Autodesk Inventor part; units mm, degrees
(part 2 of 3)
  spline S109 degree 2 poles (-64.4838, -130.0747) (-64.4838, -130.0909) (-64.4903, -130.1136) knots 0 0 0 1 1 1
  line L121 (-64.4903, -130.1136) -> (-65.1883, -133.2532)
  spline S110 degree 2 poles (-65.1883, -133.2532) (-65.2175, -133.3994) (-65.3604, -133.3994) knots 0 0 0 1 1 1
  spline S111 degree 2 poles (-65.3604, -133.3994) (-65.4838, -133.3994) (-65.5357, -133.2468) knots 0 0 0 1 1 1
  line L122 (-65.5357, -133.2468) -> (-66.0584, -131.6753)
  line L123 (-66.0584, -131.6753) -> (-66.5812, -133.2468)
  spline S112 degree 2 poles (-66.5812, -133.2468) (-66.6331, -133.3994) (-66.7597, -133.3994) knots 0 0 0 1 1 1
  spline S113 degree 2 poles (-66.7597, -133.3994) (-66.8961, -133.3994) (-66.9318, -133.2468) knots 0 0 0 1 1 1
  line L124 (-66.9318, -133.2468) -> (-67.6299, -130.1136)
  spline S114 degree 2 poles (-67.6299, -130.1136) (-67.6331, -130.0909) (-67.6331, -130.0747) knots 0 0 0 1 1 1
  spline S115 degree 2 poles (-67.6331, -130.0747) (-67.6331, -129.8994) (-67.4578, -129.8994) knots 0 0 0 1 1 1
  spline S116 degree 2 poles (-67.4578, -129.8994) (-67.3182, -129.8994) (-67.2857, -130.0357) knots 0 0 0 1 1 1
  line L125 (-67.2857, -130.0357) -> (-66.724, -132.5714)
  line L126 (-66.724, -132.5714) -> (-66.2305, -131.0942)
  spline S117 degree 2 poles (-66.2305, -131.0942) (-66.1851, -130.9513) (-66.0584, -130.9513) knots 0 0 0 1 1 1
  spline S118 degree 2 poles (-66.0584, -130.9513) (-65.9318, -130.9513) (-65.8831, -131.0942) knots 0 0 0 1 1 1
  line L127 (-65.8831, -131.0942) -> (-65.3929, -132.5682)
  spline S119 degree 2 poles (-62.9123, -133.3994) (-63.276, -133.3994) (-63.7857, -132.8864) (-63.7857, -132.5227) knots 0 0 0 1 2 2 2
  line L128 (-63.7857, -132.5227) -> (-63.7857, -132.1753)
  spline S120 degree 2 poles (-63.7857, -132.1753) (-63.7857, -131.7403) (-63.4351, -131.474) knots 0 0 0 1 1 1
  spline S121 degree 2 poles (-63.4351, -131.474) (-63.7857, -131.2078) (-63.7857, -130.7727) knots 0 0 0 1 1 1
  spline S122 degree 2 poles (-63.7857, -130.7727) (-63.7857, -130.4123) (-63.276, -129.8994) (-62.9123, -129.8994) knots 0 0 0 1 2 2 2
  spline S123 degree 2 poles (-62.9123, -129.8994) (-62.5487, -129.8994) (-62.039, -130.4123) (-62.039, -130.7727) knots 0 0 0 1 2 2 2
  spline S124 degree 2 poles (-62.039, -130.7727) (-62.039, -131.2078) (-62.3896, -131.474) knots 0 0 0 1 1 1
  spline S125 degree 2 poles (-62.3896, -131.474) (-62.1364, -131.6656) (-62.0714, -131.9448) knots 0 0 0 1 1 1
  spline S126 degree 2 poles (-62.0714, -131.9448) (-62.039, -132.0844) (-62.039, -132.5227) knots 0 0 0 1 1 1
  spline S127 degree 2 poles (-62.039, -132.5227) (-62.039, -132.8864) (-62.5487, -133.3994) (-62.9123, -133.3994) knots 0 0 0 1 2 2 2
  spline S128 degree 2 poles (-62.9123, -133.0487) (-62.6948, -133.0487) (-62.3896, -132.7435) (-62.3896, -132.5227) knots 0 0 0 1 2 2 2
  line L129 (-62.3896, -132.5227) -> (-62.3896, -132.1753)
  spline S129 degree 2 poles (-62.3896, -132.1753) (-62.3896, -131.9578) (-62.6948, -131.6494) (-62.9123, -131.6494) knots 0 0 0 1 2 2 2
  spline S130 degree 2 poles (-62.9123, -131.6494) (-63.1299, -131.6494) (-63.4351, -131.9545) (-63.4351, -132.1753) knots 0 0 0 1 2 2 2
  line L130 (-63.4351, -132.1753) -> (-63.4351, -132.5227)
  spline S131 degree 2 poles (-63.4351, -132.5227) (-63.4351, -132.7435) (-63.1299, -133.0487) (-62.9123, -133.0487) knots 0 0 0 1 2 2 2
  spline S132 degree 2 poles (-62.9123, -131.2987) (-62.6948, -131.2987) (-62.3896, -130.9968) (-62.3896, -130.776) knots 0 0 0 1 2 2 2
  spline S133 degree 2 poles (-62.3896, -130.776) (-62.3896, -130.5584) (-62.6948, -130.25) (-62.9123, -130.25) knots 0 0 0 1 2 2 2
  spline S134 degree 2 poles (-62.9123, -130.25) (-63.1299, -130.25) (-63.4351, -130.5552) (-63.4351, -130.776) knots 0 0 0 1 2 2 2
  spline S135 degree 2 poles (-63.4351, -130.776) (-63.4351, -130.9968) (-63.1299, -131.2987) (-62.9123, -131.2987) knots 0 0 0 1 2 2 2
  spline S136 degree 2 poles (-60.8117, -133.3994) (-60.8799, -133.3994) (-60.987, -133.2922) (-60.987, -133.224) knots 0 0 0 1 2 2 2
  spline S137 degree 2 poles (-60.987, -133.224) (-60.987, -133.1039) (-60.8994, -133.0747) knots 0 0 0 1 1 1
  spline S138 degree 2 poles (-60.8994, -133.0747) (-60.711, -133.0097) (-60.5844, -132.9286) knots 0 0 0 1 1 1
  spline S139 degree 2 poles (-60.5844, -132.9286) (-60.0195, -132.5617) (-59.9545, -132) knots 0 0 0 1 1 1
  line L131 (-59.9545, -132) -> (-60.4643, -132)
  spline S140 degree 2 poles (-60.4643, -132) (-60.8279, -132) (-61.3377, -131.487) (-61.3377, -131.1234) knots 0 0 0 1 2 2 2
  line L132 (-61.3377, -131.1234) -> (-61.3377, -130.776)
  spline S141 degree 2 poles (-61.3377, -130.776) (-61.3377, -130.4123) (-60.8279, -129.8994) (-60.4643, -129.8994) knots 0 0 0 1 2 2 2
  spline S142 degree 2 poles (-60.4643, -129.8994) (-60.1006, -129.8994) (-59.5909, -130.4058) (-59.5909, -130.7695) knots 0 0 0 1 2 2 2
  line L133 (-59.5909, -130.7695) -> (-59.5909, -131.8247)
  spline S143 degree 2 poles (-59.5909, -131.8247) (-59.5909, -132.7143) (-60.4188, -133.2338) knots 0 0 0 1 1 1
  spline S144 degree 2 poles (-60.4188, -133.2338) (-60.6851, -133.3994) (-60.8117, -133.3994) knots 0 0 0 1 1 1
  line L134 (-59.9416, -131.6494) -> (-59.9416, -130.776)
  spline S145 degree 2 poles (-59.9416, -130.776) (-59.9416, -130.5584) (-60.2468, -130.25) (-60.4643, -130.25) knots 0 0 0 1 2 2 2
  spline S146 degree 2 poles (-60.4643, -130.25) (-60.6818, -130.25) (-60.987, -130.5584) (-60.987, -130.776) knots 0 0 0 1 2 2 2
  line L135 (-60.987, -130.776) -> (-60.987, -131.1234)
  spline S147 degree 2 poles (-60.987, -131.1234) (-60.987, -131.3442) (-60.6818, -131.6494) (-60.4643, -131.6494) knots 0 0 0 1 2 2 2
  line L136 (-60.4643, -131.6494) -> (-59.9416, -131.6494)
  spline S148 degree 2 poles (-57.1429, -131.6494) (-57.1429, -132.276) (-57.2955, -132.7305) knots 0 0 0 1 1 1
  spline S149 degree 2 poles (-57.2955, -132.7305) (-57.5227, -133.3994) (-58.0162, -133.3994) knots 0 0 0 1 1 1
  spline S150 degree 2 poles (-58.0162, -133.3994) (-58.5097, -133.3994) (-58.737, -132.7338) knots 0 0 0 1 1 1
  spline S151 degree 2 poles (-58.737, -132.7338) (-58.8896, -132.2792) (-58.8896, -131.6494) knots 0 0 0 1 1 1
  spline S152 degree 2 poles (-58.8896, -131.6494) (-58.8896, -131.0195) (-58.737, -130.5649) knots 0 0 0 1 1 1
  spline S153 degree 2 poles (-58.737, -130.5649) (-58.5097, -129.8994) (-58.0162, -129.8994) knots 0 0 0 1 1 1
  spline S154 degree 2 poles (-58.0162, -129.8994) (-57.5227, -129.8994) (-57.2955, -130.5682) knots 0 0 0 1 1 1
  spline S155 degree 2 poles (-57.2955, -130.5682) (-57.1429, -131.0227) (-57.1429, -131.6494) knots 0 0 0 1 1 1
  spline S156 degree 2 poles (-57.4935, -131.6494) (-57.4935, -131.2143) (-57.5844, -130.8312) knots 0 0 0 1 1 1
  spline S157 degree 2 poles (-57.5844, -130.8312) (-57.7273, -130.25) (-58.0162, -130.25) knots 0 0 0 1 1 1
  spline S158 degree 2 poles (-58.0162, -130.25) (-58.3052, -130.25) (-58.4448, -130.8344) knots 0 0 0 1 1 1
  spline S159 degree 2 poles (-58.4448, -130.8344) (-58.539, -131.224) (-58.539, -131.6494) knots 0 0 0 1 1 1
  spline S160 degree 2 poles (-58.539, -131.6494) (-58.539, -132.0812) (-58.4481, -132.4675) knots 0 0 0 1 1 1
  spline S161 degree 2 poles (-58.4481, -132.4675) (-58.3052, -133.0487) (-58.0162, -133.0487) knots 0 0 0 1 1 1
  spline S162 degree 2 poles (-58.0162, -133.0487) (-57.7273, -133.0487) (-57.5844, -132.4675) knots 0 0 0 1 1 1
  spline S163 degree 2 poles (-57.5844, -132.4675) (-57.4935, -132.0812) (-57.4935, -131.6494) knots 0 0 0 1 1 1
  line L137 (-54.8669, -132.526) -> (-56.2662, -132.526)
  spline S164 degree 2 poles (-56.2662, -132.526) (-56.4416, -132.526) (-56.4416, -132.3506) knots 0 0 0 1 1 1
  spline S165 degree 2 poles (-56.4416, -132.3506) (-56.4416, -132.1753) (-56.2662, -132.1753) knots 0 0 0 1 1 1
  line L138 (-56.2662, -132.1753) -> (-54.8669, -132.1753)
  spline S166 degree 2 poles (-54.8669, -132.1753) (-54.6916, -132.1753) (-54.6916, -132.3506) knots 0 0 0 1 1 1
  spline S167 degree 2 poles (-54.6916, -132.3506) (-54.6916, -132.526) (-54.8669, -132.526) knots 0 0 0 1 1 1
  spline S168 degree 2 poles (-51.5455, -133.224) (-51.5455, -133.3994) (-51.7208, -133.3994) knots 0 0 0 1 1 1
  spline S169 degree 2 poles (-51.7208, -133.3994) (-51.8474, -133.3994) (-51.8864, -133.2792) knots 0 0 0 1 1 1
  line L139 (-51.8864, -133.2792) -> (-52.1396, -132.526)
  line L140 (-52.1396, -132.526) -> (-53.3994, -132.526)
  line L141 (-53.3994, -132.526) -> (-53.6526, -133.2792)
  spline S170 degree 2 poles (-53.6526, -133.2792) (-53.6916, -133.3994) (-53.8182, -133.3994) knots 0 0 0 1 1 1
  spline S171 degree 2 poles (-53.8182, -133.3994) (-53.9935, -133.3994) (-53.9935, -133.224) knots 0 0 0 1 1 1
  spline S172 degree 2 poles (-53.9935, -133.224) (-53.9935, -133.1916) (-53.987, -133.1688) knots 0 0 0 1 1 1
  line L142 (-53.987, -133.1688) -> (-52.9448, -130.039)
  spline S173 degree 2 poles (-52.9448, -130.039) (-52.8961, -129.8994) (-52.7695, -129.8994) knots 0 0 0 1 1 1
  spline S174 degree 2 poles (-52.7695, -129.8994) (-52.6429, -129.8994) (-52.5974, -130.0357) knots 0 0 0 1 1 1
  line L143 (-52.5974, -130.0357) -> (-51.5519, -133.1688)
  spline S175 degree 2 poles (-51.5519, -133.1688) (-51.5455, -133.1916) (-51.5455, -133.224) knots 0 0 0 1 1 1
  line L144 (-52.7695, -130.6331) -> (-53.2825, -132.1753)
  line L145 (-53.2825, -132.1753) -> (-52.2565, -132.1753)
  line L146 (-52.2565, -132.1753) -> (-52.7695, -130.6331)
  spline S176 degree 2 poles (-46.9968, -131.6494) (-46.9968, -132.276) (-47.1494, -132.7305) knots 0 0 0 1 1 1
  spline S177 degree 2 poles (-47.1494, -132.7305) (-47.3766, -133.3994) (-47.8701, -133.3994) knots 0 0 0 1 1 1
  spline S178 degree 2 poles (-47.8701, -133.3994) (-48.3636, -133.3994) (-48.5909, -132.7338) knots 0 0 0 1 1 1
  spline S179 degree 2 poles (-48.5909, -132.7338) (-48.7435, -132.2792) (-48.7435, -131.6494) knots 0 0 0 1 1 1
  spline S180 degree 2 poles (-48.7435, -131.6494) (-48.7435, -131.0195) (-48.5909, -130.5649) knots 0 0 0 1 1 1
  spline S181 degree 2 poles (-48.5909, -130.5649) (-48.3636, -129.8994) (-47.8701, -129.8994) knots 0 0 0 1 1 1
  spline S182 degree 2 poles (-47.8701, -129.8994) (-47.3766, -129.8994) (-47.1494, -130.5682) knots 0 0 0 1 1 1
  spline S183 degree 2 poles (-47.1494, -130.5682) (-46.9968, -131.0227) (-46.9968, -131.6494) knots 0 0 0 1 1 1
  spline S184 degree 2 poles (-47.3474, -131.6494) (-47.3474, -131.2143) (-47.4383, -130.8312) knots 0 0 0 1 1 1
  spline S185 degree 2 poles (-47.4383, -130.8312) (-47.5812, -130.25) (-47.8701, -130.25) knots 0 0 0 1 1 1
  spline S186 degree 2 poles (-47.8701, -130.25) (-48.1591, -130.25) (-48.2987, -130.8344) knots 0 0 0 1 1 1
  spline S187 degree 2 poles (-48.2987, -130.8344) (-48.3929, -131.224) (-48.3929, -131.6494) knots 0 0 0 1 1 1
  spline S188 degree 2 poles (-48.3929, -131.6494) (-48.3929, -132.0812) (-48.3019, -132.4675) knots 0 0 0 1 1 1
  spline S189 degree 2 poles (-48.3019, -132.4675) (-48.1591, -133.0487) (-47.8701, -133.0487) knots 0 0 0 1 1 1
  spline S190 degree 2 poles (-47.8701, -133.0487) (-47.5812, -133.0487) (-47.4383, -132.4675) knots 0 0 0 1 1 1
  spline S191 degree 2 poles (-47.4383, -132.4675) (-47.3474, -132.0812) (-47.3474, -131.6494) knots 0 0 0 1 1 1
  spline S192 degree 2 poles (-45.4221, -133.3994) (-45.7857, -133.3994) (-46.2955, -132.8864) (-46.2955, -132.5227) knots 0 0 0 1 2 2 2
  line L147 (-46.2955, -132.5227) -> (-46.2955, -132.1753)
  spline S193 degree 2 poles (-46.2955, -132.1753) (-46.2955, -131.7403) (-45.9448, -131.474) knots 0 0 0 1 1 1
  spline S194 degree 2 poles (-45.9448, -131.474) (-46.2955, -131.2078) (-46.2955, -130.7727) knots 0 0 0 1 1 1
  spline S195 degree 2 poles (-46.2955, -130.7727) (-46.2955, -130.4123) (-45.7857, -129.8994) (-45.4221, -129.8994) knots 0 0 0 1 2 2 2
  spline S196 degree 2 poles (-45.4221, -129.8994) (-45.0584, -129.8994) (-44.5487, -130.4123) (-44.5487, -130.7727) knots 0 0 0 1 2 2 2
  spline S197 degree 2 poles (-44.5487, -130.7727) (-44.5487, -131.2078) (-44.8994, -131.474) knots 0 0 0 1 1 1
  spline S198 degree 2 poles (-44.8994, -131.474) (-44.6461, -131.6656) (-44.5812, -131.9448) knots 0 0 0 1 1 1
  spline S199 degree 2 poles (-44.5812, -131.9448) (-44.5487, -132.0844) (-44.5487, -132.5227) knots 0 0 0 1 1 1
  spline S200 degree 2 poles (-44.5487, -132.5227) (-44.5487, -132.8864) (-45.0584, -133.3994) (-45.4221, -133.3994) knots 0 0 0 1 2 2 2
  spline S201 degree 2 poles (-45.4221, -133.0487) (-45.2045, -133.0487) (-44.8994, -132.7435) (-44.8994, -132.5227) knots 0 0 0 1 2 2 2
  line L148 (-44.8994, -132.5227) -> (-44.8994, -132.1753)
  spline S202 degree 2 poles (-44.8994, -132.1753) (-44.8994, -131.9578) (-45.2045, -131.6494) (-45.4221, -131.6494) knots 0 0 0 1 2 2 2
  spline S203 degree 2 poles (-45.4221, -131.6494) (-45.6396, -131.6494) (-45.9448, -131.9545) (-45.9448, -132.1753) knots 0 0 0 1 2 2 2
  line L149 (-45.9448, -132.1753) -> (-45.9448, -132.5227)
  spline S204 degree 2 poles (-45.9448, -132.5227) (-45.9448, -132.7435) (-45.6396, -133.0487) (-45.4221, -133.0487) knots 0 0 0 1 2 2 2
  spline S205 degree 2 poles (-45.4221, -131.2987) (-45.2045, -131.2987) (-44.8994, -130.9968) (-44.8994, -130.776) knots 0 0 0 1 2 2 2
  spline S206 degree 2 poles (-44.8994, -130.776) (-44.8994, -130.5584) (-45.2045, -130.25) (-45.4221, -130.25) knots 0 0 0 1 2 2 2
  spline S207 degree 2 poles (-45.4221, -130.25) (-45.6396, -130.25) (-45.9448, -130.5552) (-45.9448, -130.776) knots 0 0 0 1 2 2 2
  spline S208 degree 2 poles (-45.9448, -130.776) (-45.9448, -130.9968) (-45.6396, -131.2987) (-45.4221, -131.2987) knots 0 0 0 1 2 2 2
  spline S209 degree 2 poles (-43.8474, -133.0487) (-43.8474, -132.8734) (-43.6721, -132.8734) knots 0 0 0 1 1 1
  spline S210 degree 2 poles (-43.6721, -132.8734) (-43.4968, -132.8734) (-43.4968, -133.0487) knots 0 0 0 1 1 1
  line L150 (-43.4968, -133.0487) -> (-43.4968, -133.224)
  spline S211 degree 2 poles (-43.4968, -133.224) (-43.4968, -133.3994) (-43.6721, -133.3994) knots 0 0 0 1 1 1
  spline S212 degree 2 poles (-43.6721, -133.3994) (-43.8474, -133.3994) (-43.8474, -133.224) knots 0 0 0 1 1 1
  line L151 (-43.8474, -133.224) -> (-43.8474, -133.0487)
  spline S213 degree 2 poles (-41.9253, -129.8994) (-41.5617, -129.8994) (-41.0487, -130.4123) (-41.0487, -130.7727) knots 0 0 0 1 2 2 2
  spline S214 degree 2 poles (-41.0487, -130.7727) (-41.0487, -131.0227) (-41.2078, -131.2792) knots 0 0 0 1 1 1
  line L152 (-41.2078, -131.2792) -> (-42.3117, -133.0487)
  line L153 (-42.3117, -133.0487) -> (-41.224, -133.0487)
  spline S215 degree 2 poles (-41.224, -133.0487) (-41.0487, -133.0487) (-41.0487, -133.224) knots 0 0 0 1 1 1
  spline S216 degree 2 poles (-41.0487, -133.224) (-41.0487, -133.3994) (-41.224, -133.3994) knots 0 0 0 1 1 1
  line L154 (-41.224, -133.3994) -> (-42.6234, -133.3994)
  spline S217 degree 2 poles (-42.6234, -133.3994) (-42.7987, -133.3994) (-42.7987, -133.224) knots 0 0 0 1 1 1
  spline S218 degree 2 poles (-42.7987, -133.224) (-42.7987, -133.1721) (-42.7695, -133.1234) knots 0 0 0 1 1 1
  line L155 (-42.7695, -133.1234) -> (-41.487, -131.0649)
  spline S219 degree 2 poles (-41.487, -131.0649) (-41.3994, -130.9221) (-41.3994, -130.776) knots 0 0 0 1 1 1
  spline S220 degree 2 poles (-41.3994, -130.776) (-41.3994, -130.5584) (-41.7078, -130.25) (-41.9253, -130.25) knots 0 0 0 1 2 2 2
  spline S221 degree 2 poles (-41.9253, -130.25) (-42.2208, -130.25) (-42.474, -130.6916) knots 0 0 0 1 1 1
  spline S222 degree 2 poles (-42.474, -130.6916) (-42.5227, -130.776) (-42.6234, -130.776) knots 0 0 0 1 1 1
  spline S223 degree 2 poles (-42.6234, -130.776) (-42.7987, -130.776) (-42.7987, -130.6006) knots 0 0 0 1 1 1
  spline S224 degree 2 poles (-42.7987, -130.6006) (-42.7987, -130.5617) (-42.7825, -130.5292) knots 0 0 0 1 1 1
  spline S225 degree 2 poles (-42.7825, -130.5292) (-42.4578, -129.8994) (-41.9253, -129.8994) knots 0 0 0 1 1 1
  line L156 (-40.3506, -131.474) -> (-40.3506, -130.0747)
  spline S226 degree 2 poles (-40.3506, -130.0747) (-40.3506, -129.8994) (-40.1753, -129.8994) knots 0 0 0 1 1 1
  line L157 (-40.1753, -129.8994) -> (-38.9545, -129.8994)
  spline S227 degree 2 poles (-38.9545, -129.8994) (-38.7792, -129.8994) (-38.7792, -130.0747) knots 0 0 0 1 1 1
  spline S228 degree 2 poles (-38.7792, -130.0747) (-38.7792, -130.25) (-38.9545, -130.25) knots 0 0 0 1 1 1
  line L158 (-38.9545, -130.25) -> (-40, -130.25)
  line L159 (-40, -130.25) -> (-40, -131.2987)
  line L160 (-40, -131.2987) -> (-39.4773, -131.2987)
  spline S229 degree 2 poles (-39.4773, -131.2987) (-39.1136, -131.2987) (-38.6039, -131.8117) (-38.6039, -132.1753) knots 0 0 0 1 2 2 2
  line L161 (-38.6039, -132.1753) -> (-38.6039, -132.5227)
  spline S230 degree 2 poles (-38.6039, -132.5227) (-38.6039, -132.8864) (-39.1169, -133.3994) (-39.4773, -133.3994) knots 0 0 0 1 2 2 2
  line L162 (-39.4773, -133.3994) -> (-40.1753, -133.3994)
  spline S231 degree 2 poles (-40.1753, -133.3994) (-40.3506, -133.3994) (-40.3506, -133.224) knots 0 0 0 1 1 1
  spline S232 degree 2 poles (-40.3506, -133.224) (-40.3506, -133.0487) (-40.1753, -133.0487) knots 0 0 0 1 1 1
  line L163 (-40.1753, -133.0487) -> (-39.4773, -133.0487)
  spline S233 degree 2 poles (-39.4773, -133.0487) (-39.2597, -133.0487) (-38.9545, -132.7435) (-38.9545, -132.5227) knots 0 0 0 1 2 2 2
  line L164 (-38.9545, -132.5227) -> (-38.9545, -132.1753)
  spline S234 degree 2 poles (-38.9545, -132.1753) (-38.9545, -131.9578) (-39.2597, -131.6494) (-39.4773, -131.6494) knots 0 0 0 1 2 2 2
  line L165 (-39.4773, -131.6494) -> (-40.1753, -131.6494)
  spline S235 degree 2 poles (-40.1753, -131.6494) (-40.3506, -131.6494) (-40.3506, -131.474) knots 0 0 0 1 1 1
  spline S236 degree 2 poles (55.6313, -129.1584) (55.6313, -129) (55.792, -129) knots 0 0 0 1 1 1
  line L166 (55.792, -129) -> (56.5174, -129)
  spline S237 degree 2 poles (56.5174, -129) (56.7906, -129) (57.1625, -129.3742) (57.1625, -129.6428) knots 0 0 0 1 2 2 2
  line L167 (57.1625, -129.6428) -> (57.1625, -130.8572)
  spline S238 degree 2 poles (57.1625, -130.8572) (57.1625, -131.1258) (56.786, -131.5023) (56.5174, -131.5023) knots 0 0 0 1 2 2 2
  line L168 (56.5174, -131.5023) -> (55.792, -131.5023)
  spline S239 degree 2 poles (55.792, -131.5023) (55.6313, -131.5023) (55.6313, -131.3416) knots 0 0 0 1 1 1
  line L169 (55.6313, -131.3416) -> (55.6313, -129.1584)
  line L170 (55.9527, -129.3191) -> (55.9527, -131.1832)
  line L171 (55.9527, -131.1832) -> (56.5174, -131.1832)
  spline S240 degree 2 poles (56.5174, -131.1832) (56.6506, -131.1832) (56.8411, -130.9927) (56.8411, -130.8572) knots 0 0 0 1 2 2 2
  line L172 (56.8411, -130.8572) -> (56.8411, -129.6428)
  spline S241 degree 2 poles (56.8411, -129.6428) (56.8411, -129.5096) (56.6506, -129.3191) (56.5174, -129.3191) knots 0 0 0 1 2 2 2
  line L173 (56.5174, -129.3191) -> (55.9527, -129.3191)
  line L174 (57.6102, -131.3416) -> (57.6102, -129.1584)
  spline S242 degree 2 poles (57.6102, -129.1584) (57.6102, -129) (57.7709, -129) knots 0 0 0 1 1 1
  line L175 (57.7709, -129) -> (58.742, -129)
  spline S243 degree 2 poles (58.742, -129) (58.9027, -129) (58.9027, -129.1584) knots 0 0 0 1 1 1
  spline S244 degree 2 poles (58.9027, -129.1584) (58.9027, -129.3191) (58.742, -129.3191) knots 0 0 0 1 1 1
  line L176 (58.742, -129.3191) -> (57.9316, -129.3191)
  line L177 (57.9316, -129.3191) -> (57.9316, -129.9711)
  line L178 (57.9316, -129.9711) -> (58.4986, -129.9711)
  spline S245 degree 2 poles (58.4986, -129.9711) (58.6593, -129.9711) (58.6593, -130.1295) knots 0 0 0 1 1 1
  spline S246 degree 2 poles (58.6593, -130.1295) (58.6593, -130.2902) (58.4986, -130.2902) knots 0 0 0 1 1 1
  line L179 (58.4986, -130.2902) -> (57.9316, -130.2902)
  line L180 (57.9316, -130.2902) -> (57.9316, -131.1832)
  line L181 (57.9316, -131.1832) -> (58.742, -131.1832)
  spline S247 degree 2 poles (58.742, -131.1832) (58.9027, -131.1832) (58.9027, -131.3416) knots 0 0 0 1 1 1
  spline S248 degree 2 poles (58.9027, -131.3416) (58.9027, -131.5023) (58.742, -131.5023) knots 0 0 0 1 1 1
  line L182 (58.742, -131.5023) -> (57.7709, -131.5023)
  spline S249 degree 2 poles (57.7709, -131.5023) (57.6102, -131.5023) (57.6102, -131.3416) knots 0 0 0 1 1 1
  spline S250 degree 2 poles (59.3434, -129.1607) (59.3434, -129.0023) (59.5041, -129.0023) knots 0 0 0 1 1 1
  spline S251 degree 2 poles (59.5041, -129.0023) (59.6648, -129.0023) (59.6648, -129.1607) knots 0 0 0 1 1 1
  line L183 (59.6648, -129.1607) -> (59.6648, -131.1832)
  line L184 (59.6648, -131.1832) -> (60.4752, -131.1832)
  spline S252 degree 2 poles (60.4752, -131.1832) (60.6359, -131.1832) (60.6359, -131.3416) knots 0 0 0 1 1 1
  spline S253 degree 2 poles (60.6359, -131.3416) (60.6359, -131.5023) (60.4752, -131.5023) knots 0 0 0 1 1 1
  line L185 (60.4752, -131.5023) -> (59.5041, -131.5023)
  spline S254 degree 2 poles (59.5041, -131.5023) (59.3434, -131.5023) (59.3434, -131.3416) knots 0 0 0 1 1 1
  line L186 (59.3434, -131.3416) -> (59.3434, -129.1607)
  spline S255 degree 2 poles (61.079, -129.1584) (61.079, -129) (61.2397, -129) knots 0 0 0 1 1 1
  line L187 (61.2397, -129) -> (62.4518, -129)
  spline S256 degree 2 poles (62.4518, -129) (62.6125, -129) (62.6125, -129.1584) knots 0 0 0 1 1 1
  spline S257 degree 2 poles (62.6125, -129.1584) (62.6125, -129.3191) (62.4518, -129.3191) knots 0 0 0 1 1 1
  line L188 (62.4518, -129.3191) -> (62.0064, -129.3191)
  line L189 (62.0064, -129.3191) -> (62.0064, -131.3416)
  spline S258 degree 2 poles (62.0064, -131.3416) (62.0064, -131.5023) (61.8457, -131.5023) knots 0 0 0 1 1 1
  spline S259 degree 2 poles (61.8457, -131.5023) (61.685, -131.5023) (61.685, -131.3416) knots 0 0 0 1 1 1
  line L190 (61.685, -131.3416) -> (61.685, -129.3191)
  line L191 (61.685, -129.3191) -> (61.2397, -129.3191)
  spline S260 degree 2 poles (61.2397, -129.3191) (61.079, -129.3191) (61.079, -129.1584) knots 0 0 0 1 1 1
  spline S261 degree 2 poles (64.8347, -131.3416) (64.8347, -131.5023) (64.674, -131.5023) knots 0 0 0 1 1 1
  spline S262 degree 2 poles (64.674, -131.5023) (64.5569, -131.5023) (64.5225, -131.3944) knots 0 0 0 1 1 1
  line L192 (64.5225, -131.3944) -> (64.3549, -130.8962)
  line L193 (64.3549, -130.8962) -> (63.5376, -130.8962)
  line L194 (63.5376, -130.8962) -> (63.3724, -131.3944)
  spline S263 degree 2 poles (63.3724, -131.3944) (63.3356, -131.5023) (63.2185, -131.5023) knots 0 0 0 1 1 1
  spline S264 degree 2 poles (63.2185, -131.5023) (63.0601, -131.5023) (63.0601, -131.3416) knots 0 0 0 1 1 1
  spline S265 degree 2 poles (63.0601, -131.3416) (63.0601, -131.314) (63.067, -131.2911) knots 0 0 0 1 1 1
  line L195 (63.067, -131.2911) -> (63.7879, -129.124)
  spline S266 degree 2 poles (63.7879, -129.124) (63.8292, -129.0023) (63.9463, -129.0023) knots 0 0 0 1 1 1
  spline S267 degree 2 poles (63.9463, -129.0023) (64.0634, -129.0023) (64.1024, -129.1217) knots 0 0 0 1 1 1
  line L196 (64.1024, -129.1217) -> (64.8278, -131.2911)
  spline S268 degree 2 poles (64.8278, -131.2911) (64.8347, -131.3163) (64.8347, -131.3416) knots 0 0 0 1 1 1
  line L197 (63.9463, -129.5831) -> (63.6295, -130.5771)
  line L198 (63.6295, -130.5771) -> (64.2654, -130.5771)
  line L199 (64.2654, -130.5771) -> (63.9463, -129.5831)
  spline S269 degree 2 poles (68.3081, -130.8572) (68.3081, -131.1235) (67.9293, -131.5023) (67.663, -131.5023) knots 0 0 0 1 2 2 2
  spline S270 degree 2 poles (67.663, -131.5023) (67.2016, -131.5023) (66.8457, -131.2291) knots 0 0 0 1 1 1
  spline S271 degree 2 poles (66.8457, -131.2291) (66.7769, -131.1763) (66.7769, -131.0983) knots 0 0 0 1 1 1
  spline S272 degree 2 poles (66.7769, -131.0983) (66.7769, -131.034) (66.871, -130.9399) (66.9376, -130.9399) knots 0 0 0 1 2 2 2
  spline S273 degree 2 poles (66.9376, -130.9399) (66.9766, -130.9399) (67.0248, -130.9674) knots 0 0 0 1 1 1
  spline S274 degree 2 poles (67.0248, -130.9674) (67.1304, -131.0317) (67.3577, -131.135) knots 0 0 0 1 1 1
  spline S275 degree 2 poles (67.3577, -131.135) (67.4931, -131.1832) (67.663, -131.1832) knots 0 0 0 1 1 1
  spline S276 degree 2 poles (67.663, -131.1832) (67.7961, -131.1832) (67.9867, -130.9927) (67.9867, -130.8549) knots 0 0 0 1 2 2 2
  spline S277 degree 2 poles (67.9867, -130.8549) (67.9867, -130.6575) (67.8627, -130.5702) knots 0 0 0 1 1 1
  line L200 (67.8627, -130.5702) -> (67.1258, -130.2167)
  spline S278 degree 2 poles (67.1258, -130.2167) (66.7769, -130.0376) (66.7769, -129.6428) knots 0 0 0 1 1 1
  spline S279 degree 2 poles (66.7769, -129.6428) (66.7769, -129.3788) (67.1534, -129) (67.4219, -129) knots 0 0 0 1 2 2 2
  spline S280 degree 2 poles (67.4219, -129) (67.8604, -129) (68.0946, -129.1377) knots 0 0 0 1 1 1
  spline S281 degree 2 poles (68.0946, -129.1377) (68.1864, -129.1928) (68.1864, -129.2801) knots 0 0 0 1 1 1
  spline S282 degree 2 poles (68.1864, -129.2801) (68.1864, -129.3466) (68.0923, -129.4408) (68.0257, -129.4408) knots 0 0 0 1 2 2 2
  spline S283 degree 2 poles (68.0257, -129.4408) (67.9982, -129.4408) (67.9591, -129.4247) knots 0 0 0 1 1 1
  spline S284 degree 2 poles (67.9591, -129.4247) (67.6882, -129.3191) (67.4219, -129.3191) knots 0 0 0 1 1 1
  spline S285 degree 2 poles (67.4219, -129.3191) (67.2888, -129.3191) (67.0983, -129.5096) (67.0983, -129.6428) knots 0 0 0 1 2 2 2
  spline S286 degree 2 poles (67.0983, -129.6428) (67.0983, -129.8448) (67.2176, -129.9275) knots 0 0 0 1 1 1
  line L201 (67.2176, -129.9275) -> (67.9545, -130.2833)
  spline S287 degree 2 poles (67.9545, -130.2833) (68.3081, -130.4669) (68.3081, -130.8572) knots 0 0 0 1 1 1
  spline S288 degree 2 poles (70.2893, -130.7355) (70.2893, -131.0523) (69.8416, -131.5023) (69.5248, -131.5023) knots 0 0 0 1 2 2 2
  spline S289 degree 2 poles (69.5248, -131.5023) (69.2057, -131.5023) (68.758, -131.0546) (68.758, -130.7355) knots 0 0 0 1 2 2 2
  line L202 (68.758, -130.7355) -> (68.758, -129.7645)
  spline S290 degree 2 poles (68.758, -129.7645) (68.758, -129.4477) (69.2057, -129) (69.5248, -129) knots 0 0 0 1 2 2 2
  spline S291 degree 2 poles (69.5248, -129) (69.8439, -129) (70.2893, -129.4477) (70.2893, -129.7645) knots 0 0 0 1 2 2 2
  line L203 (70.2893, -129.7645) -> (70.2893, -130.7355)
  line L204 (69.9679, -130.7355) -> (69.9679, -129.7645)
  spline S292 degree 2 poles (69.9679, -129.7645) (69.9679, -129.5785) (69.7107, -129.3191) (69.5248, -129.3191) knots 0 0 0 1 2 2 2
  spline S293 degree 2 poles (69.5248, -129.3191) (69.3365, -129.3191) (69.0794, -129.5785) (69.0794, -129.7645) knots 0 0 0 1 2 2 2
  line L205 (69.0794, -129.7645) -> (69.0794, -130.7355)
  spline S294 degree 2 poles (69.0794, -130.7355) (69.0794, -130.9238) (69.3365, -131.1832) (69.5248, -131.1832) knots 0 0 0 1 2 2 2
  spline S295 degree 2 poles (69.5248, -131.1832) (69.7107, -131.1832) (69.9679, -130.9238) (69.9679, -130.7355) knots 0 0 0 1 2 2 2
  spline S296 degree 2 poles (70.7369, -129.1607) (70.7369, -129.0023) (70.8976, -129.0023) knots 0 0 0 1 1 1
  spline S297 degree 2 poles (70.8976, -129.0023) (71.0583, -129.0023) (71.0583, -129.1607) knots 0 0 0 1 1 1
  line L206 (71.0583, -129.1607) -> (71.0583, -131.1832)
  line L207 (71.0583, -131.1832) -> (71.8687, -131.1832)
  spline S298 degree 2 poles (71.8687, -131.1832) (72.0294, -131.1832) (72.0294, -131.3416) knots 0 0 0 1 1 1
  spline S299 degree 2 poles (72.0294, -131.3416) (72.0294, -131.5023) (71.8687, -131.5023) knots 0 0 0 1 1 1
  line L208 (71.8687, -131.5023) -> (70.8976, -131.5023)
  spline S300 degree 2 poles (70.8976, -131.5023) (70.7369, -131.5023) (70.7369, -131.3416) knots 0 0 0 1 1 1
  line L209 (70.7369, -131.3416) -> (70.7369, -129.1607)
  spline S301 degree 2 poles (72.4702, -129.1607) (72.4702, -129.0023) (72.6309, -129.0023) knots 0 0 0 1 1 1
  spline S302 degree 2 poles (72.6309, -129.0023) (72.7916, -129.0023) (72.7916, -129.1607) knots 0 0 0 1 1 1
  line L210 (72.7916, -129.1607) -> (72.7916, -131.1832)
  line L211 (72.7916, -131.1832) -> (73.6019, -131.1832)
  spline S303 degree 2 poles (73.6019, -131.1832) (73.7626, -131.1832) (73.7626, -131.3416) knots 0 0 0 1 1 1
  spline S304 degree 2 poles (73.7626, -131.3416) (73.7626, -131.5023) (73.6019, -131.5023) knots 0 0 0 1 1 1
  line L212 (73.6019, -131.5023) -> (72.6309, -131.5023)
  spline S305 degree 2 poles (72.6309, -131.5023) (72.4702, -131.5023) (72.4702, -131.3416) knots 0 0 0 1 1 1
  line L213 (72.4702, -131.3416) -> (72.4702, -129.1607)
  line L214 (75.7369, -129.1607) -> (75.7369, -130.7355)
  spline S306 degree 2 poles (75.7369, -130.7355) (75.7369, -131.0546) (75.2893, -131.5023) (74.9725, -131.5023) knots 0 0 0 1 2 2 2
  spline S307 degree 2 poles (74.9725, -131.5023) (74.6534, -131.5023) (74.2057, -131.0546) (74.2057, -130.7355) knots 0 0 0 1 2 2 2
  line L215 (74.2057, -130.7355) -> (74.2057, -129.1607)
  spline S308 degree 2 poles (74.2057, -129.1607) (74.2057, -129.0023) (74.3664, -129.0023) knots 0 0 0 1 1 1
  spline S309 degree 2 poles (74.3664, -129.0023) (74.5271, -129.0023) (74.5271, -129.1607) knots 0 0 0 1 1 1
  line L216 (74.5271, -129.1607) -> (74.5271, -130.7355)
  spline S310 degree 2 poles (74.5271, -130.7355) (74.5271, -130.9238) (74.7842, -131.1832) (74.9725, -131.1832) knots 0 0 0 1 2 2 2
  spline S311 degree 2 poles (74.9725, -131.1832) (75.1584, -131.1832) (75.4155, -130.9238) (75.4155, -130.7355) knots 0 0 0 1 2 2 2
  line L217 (75.4155, -130.7355) -> (75.4155, -129.1607)
  spline S312 degree 2 poles (75.4155, -129.1607) (75.4155, -129.0023) (75.5762, -129.0023) knots 0 0 0 1 1 1
  spline S313 degree 2 poles (75.5762, -129.0023) (75.7369, -129.0023) (75.7369, -129.1607) knots 0 0 0 1 1 1
  spline S314 degree 2 poles (76.1869, -129.1584) (76.1869, -129) (76.3476, -129) knots 0 0 0 1 1 1
  line L218 (76.3476, -129) -> (77.5597, -129)
  spline S315 degree 2 poles (77.5597, -129) (77.7204, -129) (77.7204, -129.1584) knots 0 0 0 1 1 1
  spline S316 degree 2 poles (77.7204, -129.1584) (77.7204, -129.3191) (77.5597, -129.3191) knots 0 0 0 1 1 1
  line L219 (77.5597, -129.3191) -> (77.1143, -129.3191)
  line L220 (77.1143, -129.3191) -> (77.1143, -131.3416)
  spline S317 degree 2 poles (77.1143, -131.3416) (77.1143, -131.5023) (76.9536, -131.5023) knots 0 0 0 1 1 1
  spline S318 degree 2 poles (76.9536, -131.5023) (76.7929, -131.5023) (76.7929, -131.3416) knots 0 0 0 1 1 1
  line L221 (76.7929, -131.3416) -> (76.7929, -129.3191)
  line L222 (76.7929, -129.3191) -> (76.3476, -129.3191)
  spline S319 degree 2 poles (76.3476, -129.3191) (76.1869, -129.3191) (76.1869, -129.1584) knots 0 0 0 1 1 1
  spline S320 degree 2 poles (78.3264, -131.5023) (78.1657, -131.5023) (78.1657, -131.3416) knots 0 0 0 1 1 1
  line L223 (78.1657, -131.3416) -> (78.1657, -129.1607)
  spline S321 degree 2 poles (78.1657, -129.1607) (78.1657, -129.0023) (78.3264, -129.0023) knots 0 0 0 1 1 1
  spline S322 degree 2 poles (78.3264, -129.0023) (78.4871, -129.0023) (78.4871, -129.1607) knots 0 0 0 1 1 1
  line L224 (78.4871, -129.1607) -> (78.4871, -131.3416)
  spline S323 degree 2 poles (78.4871, -131.3416) (78.4871, -131.5023) (78.3264, -131.5023) knots 0 0 0 1 1 1
  spline S324 degree 2 poles (80.4431, -130.7355) (80.4431, -131.0523) (79.9954, -131.5023) (79.6786, -131.5023) knots 0 0 0 1 2 2 2
  spline S325 degree 2 poles (79.6786, -131.5023) (79.3595, -131.5023) (78.9118, -131.0546) (78.9118, -130.7355) knots 0 0 0 1 2 2 2
  line L225 (78.9118, -130.7355) -> (78.9118, -129.7645)
  spline S326 degree 2 poles (78.9118, -129.7645) (78.9118, -129.4477) (79.3595, -129) (79.6786, -129) knots 0 0 0 1 2 2 2
  spline S327 degree 2 poles (79.6786, -129) (79.9977, -129) (80.4431, -129.4477) (80.4431, -129.7645) knots 0 0 0 1 2 2 2
  line L226 (80.4431, -129.7645) -> (80.4431, -130.7355)
  line L227 (80.1217, -130.7355) -> (80.1217, -129.7645)
  spline S328 degree 2 poles (80.1217, -129.7645) (80.1217, -129.5785) (79.8646, -129.3191) (79.6786, -129.3191) knots 0 0 0 1 2 2 2
  spline S329 degree 2 poles (79.6786, -129.3191) (79.4904, -129.3191) (79.2332, -129.5785) (79.2332, -129.7645) knots 0 0 0 1 2 2 2
  line L228 (79.2332, -129.7645) -> (79.2332, -130.7355)
  spline S330 degree 2 poles (79.2332, -130.7355) (79.2332, -130.9238) (79.4904, -131.1832) (79.6786, -131.1832) knots 0 0 0 1 2 2 2
  spline S331 degree 2 poles (79.6786, -131.1832) (79.8646, -131.1832) (80.1217, -130.9238) (80.1217, -130.7355) knots 0 0 0 1 2 2 2
  line L229 (82.1028, -130.8343) -> (82.1028, -129.1607)
  spline S332 degree 2 poles (82.1028, -129.1607) (82.1028, -129.0023) (82.2635, -129.0023) knots 0 0 0 1 1 1
  spline S333 degree 2 poles (82.2635, -129.0023) (82.4242, -129.0023) (82.4242, -129.1607) knots 0 0 0 1 1 1
  line L230 (82.4242, -129.1607) -> (82.4242, -131.3416)
  spline S334 degree 2 poles (82.4242, -131.3416) (82.4242, -131.5023) (82.2635, -131.5023) knots 0 0 0 1 1 1
  spline S335 degree 2 poles (82.2635, -131.5023) (82.1648, -131.5023) (82.1212, -131.4219) knots 0 0 0 1 1 1
  line L231 (82.1212, -131.4219) -> (81.2144, -129.6657)
  line L232 (81.2144, -129.6657) -> (81.2144, -131.3416)
  spline S336 degree 2 poles (81.2144, -131.3416) (81.2144, -131.5023) (81.0537, -131.5023) knots 0 0 0 1 1 1
  spline S337 degree 2 poles (81.0537, -131.5023) (80.893, -131.5023) (80.893, -131.3416) knots 0 0 0 1 1 1
  line L233 (80.893, -131.3416) -> (80.893, -129.1607)
  spline S338 degree 2 poles (80.893, -129.1607) (80.893, -129.0023) (81.0537, -129.0023) knots 0 0 0 1 1 1
  spline S339 degree 2 poles (81.0537, -129.0023) (81.1478, -129.0023) (81.1869, -129.0712) knots 0 0 0 1 1 1
  line L234 (81.1869, -129.0712) -> (82.1028, -130.8343)
  spline S340 degree 2 poles (84.4054, -130.8572) (84.4054, -131.1235) (84.0266, -131.5023) (83.7603, -131.5023) knots 0 0 0 1 2 2 2
  spline S341 degree 2 poles (83.7603, -131.5023) (83.2989, -131.5023) (82.9431, -131.2291) knots 0 0 0 1 1 1
  spline S342 degree 2 poles (82.9431, -131.2291) (82.8742, -131.1763) (82.8742, -131.0983) knots 0 0 0 1 1 1
  spline S343 degree 2 poles (82.8742, -131.0983) (82.8742, -131.034) (82.9683, -130.9399) (83.0349, -130.9399) knots 0 0 0 1 2 2 2
  spline S344 degree 2 poles (83.0349, -130.9399) (83.0739, -130.9399) (83.1221, -130.9674) knots 0 0 0 1 1 1
  spline S345 degree 2 poles (83.1221, -130.9674) (83.2277, -131.0317) (83.455, -131.135) knots 0 0 0 1 1 1
  spline S346 degree 2 poles (83.455, -131.135) (83.5904, -131.1832) (83.7603, -131.1832) knots 0 0 0 1 1 1
  spline S347 degree 2 poles (83.7603, -131.1832) (83.8935, -131.1832) (84.084, -130.9927) (84.084, -130.8549) knots 0 0 0 1 2 2 2
  spline S348 degree 2 poles (84.084, -130.8549) (84.084, -130.6575) (83.9601, -130.5702) knots 0 0 0 1 1 1
  line L235 (83.9601, -130.5702) -> (83.2231, -130.2167)
  spline S349 degree 2 poles (83.2231, -130.2167) (82.8742, -130.0376) (82.8742, -129.6428) knots 0 0 0 1 1 1
  spline S350 degree 2 poles (82.8742, -129.6428) (82.8742, -129.3788) (83.2507, -129) (83.5193, -129) knots 0 0 0 1 2 2 2
  spline S351 degree 2 poles (83.5193, -129) (83.9578, -129) (84.1919, -129.1377) knots 0 0 0 1 1 1
  spline S352 degree 2 poles (84.1919, -129.1377) (84.2837, -129.1928) (84.2837, -129.2801) knots 0 0 0 1 1 1
  spline S353 degree 2 poles (84.2837, -129.2801) (84.2837, -129.3466) (84.1896, -129.4408) (84.123, -129.4408) knots 0 0 0 1 2 2 2
  spline S354 degree 2 poles (84.123, -129.4408) (84.0955, -129.4408) (84.0565, -129.4247) knots 0 0 0 1 1 1
  spline S355 degree 2 poles (84.0565, -129.4247) (83.7856, -129.3191) (83.5193, -129.3191) knots 0 0 0 1 1 1
  spline S356 degree 2 poles (83.5193, -129.3191) (83.3861, -129.3191) (83.1956, -129.5096) (83.1956, -129.6428) knots 0 0 0 1 2 2 2
  spline S357 degree 2 poles (83.1956, -129.6428) (83.1956, -129.8448) (83.315, -129.9275) knots 0 0 0 1 1 1
  line L236 (83.315, -129.9275) -> (84.0519, -130.2833)
  spline S358 degree 2 poles (84.0519, -130.2833) (84.4054, -130.4669) (84.4054, -130.8572) knots 0 0 0 1 1 1
  spline S359 degree 2 poles (61.5895, -134.896) (61.5138, -134.896) (61.489, -134.8244) knots 0 0 0 1 1 1
  line L237 (61.489, -134.8244) -> (61.011, -133.5227)
  spline S360 degree 2 poles (61.011, -133.5227) (61.0055, -133.509) (61.0055, -133.491) knots 0 0 0 1 1 1
  spline S361 degree 2 poles (61.0055, -133.491) (61.0055, -133.396) (61.1088, -133.396) knots 0 0 0 1 1 1
  spline S362 degree 2 poles (61.1088, -133.396) (61.1846, -133.396) (61.208, -133.4594) knots 0 0 0 1 1 1
  line L238 (61.208, -133.4594) -> (61.5895, -134.5448)
  line L239 (61.5895, -134.5448) -> (61.9711, -133.4594)
  spline S363 degree 2 poles (61.9711, -133.4594) (61.9945, -133.396) (62.0702, -133.396) knots 0 0 0 1 1 1
  spline S364 degree 2 poles (62.0702, -133.396) (62.1736, -133.396) (62.1736, -133.491) knots 0 0 0 1 1 1
  spline S365 degree 2 poles (62.1736, -133.491) (62.1736, -133.509) (62.168, -133.5227) knots 0 0 0 1 1 1
  line L240 (62.168, -133.5227) -> (61.6901, -134.8244)
  spline S366 degree 2 poles (61.6901, -134.8244) (61.6639, -134.896) (61.5895, -134.896) knots 0 0 0 1 1 1
  spline S367 degree 2 poles (62.5799, -134.896) (62.4766, -134.896) (62.4766, -134.7996) knots 0 0 0 1 1 1
  line L241 (62.4766, -134.7996) -> (62.4766, -133.491)
  spline S368 degree 2 poles (62.4766, -133.491) (62.4766, -133.396) (62.5799, -133.396) knots 0 0 0 1 1 1
  spline S369 degree 2 poles (62.5799, -133.396) (62.6832, -133.396) (62.6832, -133.491) knots 0 0 0 1 1 1
  line L242 (62.6832, -133.491) -> (62.6832, -134.7996)
  spline S370 degree 2 poles (62.6832, -134.7996) (62.6832, -134.896) (62.5799, -134.896) knots 0 0 0 1 1 1
  spline S371 degree 2 poles (63.5523, -134.896) (63.4766, -134.896) (63.4518, -134.8244) knots 0 0 0 1 1 1
  line L243 (63.4518, -134.8244) -> (62.9738, -133.5227)
  spline S372 degree 2 poles (62.9738, -133.5227) (62.9683, -133.509) (62.9683, -133.491) knots 0 0 0 1 1 1
  spline S373 degree 2 poles (62.9683, -133.491) (62.9683, -133.396) (63.0716, -133.396) knots 0 0 0 1 1 1
  spline S374 degree 2 poles (63.0716, -133.396) (63.1474, -133.396) (63.1708, -133.4594) knots 0 0 0 1 1 1
  line L244 (63.1708, -133.4594) -> (63.5523, -134.5448)
  line L245 (63.5523, -134.5448) -> (63.9339, -133.4594)
  spline S375 degree 2 poles (63.9339, -133.4594) (63.9573, -133.396) (64.0331, -133.396) knots 0 0 0 1 1 1
  spline S376 degree 2 poles (64.0331, -133.396) (64.1364, -133.396) (64.1364, -133.491) knots 0 0 0 1 1 1
  spline S377 degree 2 poles (64.1364, -133.491) (64.1364, -133.509) (64.1309, -133.5227) knots 0 0 0 1 1 1
  line L246 (64.1309, -133.5227) -> (63.6529, -134.8244)
  spline S378 degree 2 poles (63.6529, -134.8244) (63.6267, -134.896) (63.5523, -134.896) knots 0 0 0 1 1 1
  spline S379 degree 2 poles (65.6074, -134.7996) (65.6074, -134.896) (65.5041, -134.896) knots 0 0 0 1 1 1
  spline S380 degree 2 poles (65.5041, -134.896) (65.4284, -134.896) (65.405, -134.8313) knots 0 0 0 1 1 1
  line L247 (65.405, -134.8313) -> (65.2948, -134.5324)
  line L248 (65.2948, -134.5324) -> (64.7507, -134.5324)
  line L249 (64.7507, -134.5324) -> (64.6419, -134.8313)
  spline S381 degree 2 poles (64.6419, -134.8313) (64.6185, -134.896) (64.5427, -134.896) knots 0 0 0 1 1 1
  spline S382 degree 2 poles (64.5427, -134.896) (64.4394, -134.896) (64.4394, -134.7996) knots 0 0 0 1 1 1
  spline S383 degree 2 poles (64.4394, -134.7996) (64.4394, -134.7817) (64.4449, -134.7693) knots 0 0 0 1 1 1
  line L250 (64.4449, -134.7693) -> (64.9201, -133.4993)
  spline S384 degree 2 poles (64.9201, -133.4993) (64.949, -133.396) (65.0234, -133.396) knots 0 0 0 1 1 1
  spline S385 degree 2 poles (65.0234, -133.396) (65.0978, -133.396) (65.124, -133.4663) knots 0 0 0 1 1 1
  line L251 (65.124, -133.4663) -> (65.6019, -134.7693)
  spline S386 degree 2 poles (65.6019, -134.7693) (65.6074, -134.7831) (65.6074, -134.7996) knots 0 0 0 1 1 1
  line L252 (65.0234, -133.7445) -> (64.8113, -134.3409)
  line L253 (64.8113, -134.3409) -> (65.2355, -134.3409)
  line L254 (65.2355, -134.3409) -> (65.0234, -133.7445)
  spline S387 degree 2 poles (68.0592, -134.7996) (68.0592, -134.896) (67.9559, -134.896) knots 0 0 0 1 1 1
  spline S388 degree 2 poles (67.9559, -134.896) (67.8802, -134.896) (67.8567, -134.8313) knots 0 0 0 1 1 1
  line L255 (67.8567, -134.8313) -> (67.7466, -134.5324)
  line L256 (67.7466, -134.5324) -> (67.2025, -134.5324)
  line L257 (67.2025, -134.5324) -> (67.0937, -134.8313)
  spline S389 degree 2 poles (67.0937, -134.8313) (67.0702, -134.896) (66.9945, -134.896) knots 0 0 0 1 1 1
  spline S390 degree 2 poles (66.9945, -134.896) (66.8912, -134.896) (66.8912, -134.7996) knots 0 0 0 1 1 1
  spline S391 degree 2 poles (66.8912, -134.7996) (66.8912, -134.7817) (66.8967, -134.7693) knots 0 0 0 1 1 1
  line L258 (66.8967, -134.7693) -> (67.3719, -133.4993)
  spline S392 degree 2 poles (67.3719, -133.4993) (67.4008, -133.396) (67.4752, -133.396) knots 0 0 0 1 1 1
  spline S393 degree 2 poles (67.4752, -133.396) (67.5496, -133.396) (67.5758, -133.4663) knots 0 0 0 1 1 1
  line L259 (67.5758, -133.4663) -> (68.0537, -134.7693)
  spline S394 degree 2 poles (68.0537, -134.7693) (68.0592, -134.7831) (68.0592, -134.7996) knots 0 0 0 1 1 1
  line L260 (67.4752, -133.7445) -> (67.2631, -134.3409)
  line L261 (67.2631, -134.3409) -> (67.6873, -134.3409)
  line L262 (67.6873, -134.3409) -> (67.4752, -133.7445)
  spline S395 degree 2 poles (67.2121, -132.907) (67.2121, -132.8134) (67.3154, -132.8134) knots 0 0 0 1 1 1
  spline S396 degree 2 poles (67.3154, -132.8134) (67.3499, -132.8134) (67.3691, -132.8258) knots 0 0 0 1 1 1
  line L263 (67.3691, -132.8258) -> (67.6915, -133.0461)
  spline S397 degree 2 poles (67.6915, -133.0461) (67.7383, -133.0778) (67.7383, -133.126) knots 0 0 0 1 1 1
  spline S398 degree 2 poles (67.7383, -133.126) (67.7383, -133.2225) (67.635, -133.2225) knots 0 0 0 1 1 1
  spline S399 degree 2 poles (67.635, -133.2225) (67.5992, -133.2225) (67.573, -133.2032) knots 0 0 0 1 1 1
  line L264 (67.573, -133.2032) -> (67.259, -132.9897)
  spline S400 degree 2 poles (67.259, -132.9897) (67.2121, -132.958) (67.2121, -132.907) knots 0 0 0 1 1 1
  spline S401 degree 2 poles (69.4463, -134.896) (69.343, -134.896) (69.343, -134.7996) knots 0 0 0 1 1 1
  line L265 (69.343, -134.7996) -> (69.343, -133.491)
  spline S402 degree 2 poles (69.343, -133.491) (69.343, -133.396) (69.4463, -133.396) knots 0 0 0 1 1 1
  spline S403 degree 2 poles (69.4463, -133.396) (69.5496, -133.396) (69.5496, -133.491) knots 0 0 0 1 1 1
  line L266 (69.5496, -133.491) -> (69.5496, -134.7996)
  spline S404 degree 2 poles (69.5496, -134.7996) (69.5496, -134.896) (69.4463, -134.896) knots 0 0 0 1 1 1
  line L267 (70.6364, -134.4952) -> (70.6364, -133.491)
  spline S405 degree 2 poles (70.6364, -133.491) (70.6364, -133.396) (70.7397, -133.396) knots 0 0 0 1 1 1
  spline S406 degree 2 poles (70.7397, -133.396) (70.843, -133.396) (70.843, -133.491) knots 0 0 0 1 1 1
  line L268 (70.843, -133.491) -> (70.843, -134.7996)
  spline S407 degree 2 poles (70.843, -134.7996) (70.843, -134.896) (70.7397, -134.896) knots 0 0 0 1 1 1
  spline S408 degree 2 poles (70.7397, -134.896) (70.6777, -134.896) (70.6598, -134.8602) knots 0 0 0 1 1 1
  line L269 (70.6598, -134.8602) -> (70.0413, -133.7941)
  line L270 (70.0413, -133.7941) -> (70.0413, -134.7996)
  spline S409 degree 2 poles (70.0413, -134.7996) (70.0413, -134.896) (69.938, -134.896) knots 0 0 0 1 1 1
  spline S410 degree 2 poles (69.938, -134.896) (69.8347, -134.896) (69.8347, -134.7996) knots 0 0 0 1 1 1
  line L271 (69.8347, -134.7996) -> (69.8347, -133.491)
  spline S411 degree 2 poles (69.8347, -133.491) (69.8347, -133.396) (69.938, -133.396) knots 0 0 0 1 1 1
  spline S412 degree 2 poles (69.938, -133.396) (69.9986, -133.396) (70.0317, -133.4497) knots 0 0 0 1 1 1
  line L272 (70.0317, -133.4497) -> (70.6364, -134.4952)
  spline S413 degree 2 poles (72.1501, -134.436) (72.1501, -134.6274) (71.854, -134.896) (71.646, -134.896) knots 0 0 0 1 2 2 2
  spline S414 degree 2 poles (71.646, -134.896) (71.4366, -134.896) (71.1419, -134.6274) (71.1419, -134.436) knots 0 0 0 1 2 2 2
  line L273 (71.1419, -134.436) -> (71.1419, -133.8533)
  spline S415 degree 2 poles (71.1419, -133.8533) (71.1419, -133.6632) (71.4366, -133.3946) (71.646, -133.3946) knots 0 0 0 1 2 2 2
  spline S416 degree 2 poles (71.646, -133.3946) (71.8554, -133.3946) (72.1501, -133.6618) (72.1501, -133.8533) knots 0 0 0 1 2 2 2
  line L274 (72.1501, -133.8533) -> (72.1501, -134.436)
  line L275 (71.9435, -134.436) -> (71.9435, -133.8533)
  spline S417 degree 2 poles (71.9435, -133.8533) (71.9435, -133.7417) (71.7713, -133.5861) (71.646, -133.5861) knots 0 0 0 1 2 2 2
  spline S418 degree 2 poles (71.646, -133.5861) (71.5207, -133.5861) (71.3485, -133.7417) (71.3485, -133.8533) knots 0 0 0 1 2 2 2
  line L276 (71.3485, -133.8533) -> (71.3485, -134.436)
  spline S419 degree 2 poles (71.3485, -134.436) (71.3485, -134.5489) (71.5207, -134.7045) (71.646, -134.7045) knots 0 0 0 1 2 2 2
  spline S420 degree 2 poles (71.646, -134.7045) (71.7713, -134.7045) (71.9435, -134.5489) (71.9435, -134.436) knots 0 0 0 1 2 2 2
  spline S421 degree 2 poles (73.0331, -134.896) (72.9573, -134.896) (72.9325, -134.8244) knots 0 0 0 1 1 1
  line L277 (72.9325, -134.8244) -> (72.4545, -133.5227)
  spline S422 degree 2 poles (72.4545, -133.5227) (72.449, -133.509) (72.449, -133.491) knots 0 0 0 1 1 1
  spline S423 degree 2 poles (72.449, -133.491) (72.449, -133.396) (72.5523, -133.396) knots 0 0 0 1 1 1
  spline S424 degree 2 poles (72.5523, -133.396) (72.6281, -133.396) (72.6515, -133.4594) knots 0 0 0 1 1 1
  line L278 (72.6515, -133.4594) -> (73.0331, -134.5448)
  line L279 (73.0331, -134.5448) -> (73.4146, -133.4594)
  spline S425 degree 2 poles (73.4146, -133.4594) (73.438, -133.396) (73.5138, -133.396) knots 0 0 0 1 1 1
  spline S426 degree 2 poles (73.5138, -133.396) (73.6171, -133.396) (73.6171, -133.491) knots 0 0 0 1 1 1
  spline S427 degree 2 poles (73.6171, -133.491) (73.6171, -133.509) (73.6116, -133.5227) knots 0 0 0 1 1 1
  line L280 (73.6116, -133.5227) -> (73.1336, -134.8244)
  spline S428 degree 2 poles (73.1336, -134.8244) (73.1074, -134.896) (73.0331, -134.896) knots 0 0 0 1 1 1
  spline S429 degree 2 poles (75.0882, -134.7996) (75.0882, -134.896) (74.9848, -134.896) knots 0 0 0 1 1 1
  spline S430 degree 2 poles (74.9848, -134.896) (74.9091, -134.896) (74.8857, -134.8313) knots 0 0 0 1 1 1
  line L281 (74.8857, -134.8313) -> (74.7755, -134.5324)
  line L282 (74.7755, -134.5324) -> (74.2314, -134.5324)
  line L283 (74.2314, -134.5324) -> (74.1226, -134.8313)
  spline S431 degree 2 poles (74.1226, -134.8313) (74.0992, -134.896) (74.0234, -134.896) knots 0 0 0 1 1 1
  spline S432 degree 2 poles (74.0234, -134.896) (73.9201, -134.896) (73.9201, -134.7996) knots 0 0 0 1 1 1
  spline S433 degree 2 poles (73.9201, -134.7996) (73.9201, -134.7817) (73.9256, -134.7693) knots 0 0 0 1 1 1
  line L284 (73.9256, -134.7693) -> (74.4008, -133.4993)
  spline S434 degree 2 poles (74.4008, -133.4993) (74.4298, -133.396) (74.5041, -133.396) knots 0 0 0 1 1 1
  spline S435 degree 2 poles (74.5041, -133.396) (74.5785, -133.396) (74.6047, -133.4663) knots 0 0 0 1 1 1
  line L285 (74.6047, -133.4663) -> (75.0826, -134.7693)
  spline S436 degree 2 poles (75.0826, -134.7693) (75.0882, -134.7831) (75.0882, -134.7996) knots 0 0 0 1 1 1
  line L286 (74.5041, -133.7445) -> (74.292, -134.3409)
  line L287 (74.292, -134.3409) -> (74.7163, -134.3409)
  line L288 (74.7163, -134.3409) -> (74.5041, -133.7445)
  spline S437 degree 2 poles (75.7342, -135.1866) (75.6309, -135.1866) (75.6309, -135.0902) knots 0 0 0 1 1 1
  spline S438 degree 2 poles (75.6309, -135.0902) (75.6309, -135.0792) (75.6915, -134.8781) knots 0 0 0 1 1 1
  spline S439 degree 2 poles (75.6915, -134.8781) (75.5702, -134.8519) (75.3912, -134.6412) (75.3912, -134.5076) knots 0 0 0 1 2 2 2
  line L289 (75.3912, -134.5076) -> (75.3912, -133.7803)
  spline S440 degree 2 poles (75.3912, -133.7803) (75.3912, -133.6205) (75.6391, -133.3946) (75.814, -133.3946) knots 0 0 0 1 2 2 2
  line L290 (75.814, -133.3946) -> (76.135, -133.3946)
  spline S441 degree 2 poles (76.135, -133.3946) (76.2383, -133.3946) (76.2383, -133.4897) knots 0 0 0 1 1 1
  spline S442 degree 2 poles (76.2383, -133.4897) (76.2383, -133.5861) (76.135, -133.5861) knots 0 0 0 1 1 1
  line L291 (76.135, -133.5861) -> (75.814, -133.5861)
  spline S443 degree 2 poles (75.814, -133.5861) (75.6887, -133.5861) (75.6267, -133.6839) knots 0 0 0 1 1 1
  spline S444 degree 2 poles (75.6267, -133.6839) (75.5978, -133.728) (75.5978, -133.7803) knots 0 0 0 1 1 1
  line L292 (75.5978, -133.7803) -> (75.5978, -134.509)
  spline S445 degree 2 poles (75.5978, -134.509) (75.5978, -134.5888) (75.7245, -134.7045) (75.814, -134.7045) knots 0 0 0 1 2 2 2
  line L293 (75.814, -134.7045) -> (76.135, -134.7045)
  spline S446 degree 2 poles (76.135, -134.7045) (76.2383, -134.7045) (76.2383, -134.7996) knots 0 0 0 1 1 1
  spline S447 degree 2 poles (76.2383, -134.7996) (76.2383, -134.896) (76.135, -134.896) knots 0 0 0 1 1 1
  line L294 (76.135, -134.896) -> (75.8953, -134.896)
  line L295 (75.8953, -134.896) -> (75.8347, -135.115)
  spline S448 degree 2 poles (75.8347, -135.115) (75.814, -135.1866) (75.7342, -135.1866) knots 0 0 0 1 1 1
  spline S449 degree 2 poles (77.7039, -134.7996) (77.7039, -134.896) (77.6006, -134.896) knots 0 0 0 1 1 1
  spline S450 degree 2 poles (77.6006, -134.896) (77.5248, -134.896) (77.5014, -134.8313) knots 0 0 0 1 1 1
  line L296 (77.5014, -134.8313) -> (77.3912, -134.5324)
  line L297 (77.3912, -134.5324) -> (76.8471, -134.5324)
  line L298 (76.8471, -134.5324) -> (76.7383, -134.8313)
  spline S451 degree 2 poles (76.7383, -134.8313) (76.7149, -134.896) (76.6391, -134.896) knots 0 0 0 1 1 1
  spline S452 degree 2 poles (76.6391, -134.896) (76.5358, -134.896) (76.5358, -134.7996) knots 0 0 0 1 1 1
  spline S453 degree 2 poles (76.5358, -134.7996) (76.5358, -134.7817) (76.5413, -134.7693) knots 0 0 0 1 1 1
  line L299 (76.5413, -134.7693) -> (77.0165, -133.4993)